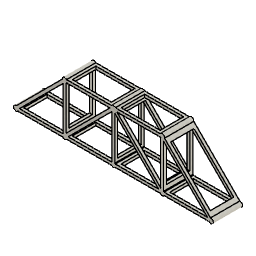
aarav (Autodesk Fusion 360 design; units mm, degrees)
Autodesk Fusion 360 part; units mm, degrees
note: some values were not read from the file. Set by a fixed rule: which sketch regions a step uses.
sketch "Sketch1" plane through (0, 0, 0) normal (0, 1, 0) x (1, 0, 0)
  circle A0 centre (-75, 0) radius 2.5
  line L0 (-75, 0) -> (25, 0) construction
  circle A1 centre (25, 0) radius 2.5
  line L1 (25, 0) -> (25, -50) construction
  line L2 (25, -50) -> (-25, -50) construction
  line L3 (-25, -50) -> (-75, 0) construction
  line L4 (25, -50) -> (-25, 0) construction
  line L5 (-25, -50) -> (-25, 0) construction
  circle A2 centre (-25, -50) radius 2.5
  circle A3 centre (25, -50) radius 2.5
  circle A4 centre (-25, 0) radius 2.5
  line L6 (-23.9393, -48.9393) -> (-73.9393, 1.0607)
  line L7 (-26.0607, -51.0607) -> (-76.0607, -1.0607)
  line L8 (25, -48.5) -> (-25, -48.5)
  line L9 (25, -51.5) -> (-25, -51.5)
  line L10 (23.5, 0) -> (23.5, -50)
  line L11 (26.5, 0) -> (26.5, -50)
  line L12 (23.9393, -51.0607) -> (-26.0607, -1.0607)
  line L13 (26.0607, -48.9393) -> (-23.9393, 1.0607)
  line L14 (-75, -1.5) -> (25, -1.5)
  line L15 (-75, 1.5) -> (25, 1.5)
  line L16 (-23.5, -50) -> (-23.5, 0)
  line L17 (-26.5, -50) -> (-26.5, 0)
  dimension "d1" = 5
  dimension "d2" = 5
  dimension "d3" = 5
  dimension "d4" = 5
  dimension "d5" = 5
  dimension "d6" = 1.5
  dimension "d7" = -1.5
  dimension "d8" = 1.5
  dimension "d9" = -1.5
  dimension "d10" = 1.5
  dimension "d11" = -1.5
  dimension "d12" = -1.5
  dimension "d13" = 1.5
  dimension "d14" = 1.5
  dimension "d15" = -1.5
  dimension "d16" = 1.5
  dimension "d17" = -1.5
  constraint coincident A0.centre L0.start
  constraint horizontal L0
  constraint coincident L0.end A1.centre
  constraint perpendicular L0 L1
  constraint perpendicular L1 L2
  constraint midpoint L0 L4.end
  constraint perpendicular L0 L5
  constraint coincident L2.end L3.start
  constraint coincident L1.end L2.start
  constraint coincident L4.end L5.end
  measures "d1" diameter of A0
  measures "d2" diameter of A1
  measures "d3" diameter of A2
  measures "d4" diameter of A3
  measures "d5" diameter of A4
extrude "Extrude1" add sketch "Sketch1" along normal blind 30 contours A0 | A0 A4 L6 L14 L15 | A0 L6 L14 | A0 A2 L6 L7 L14 L17 | A4 L14 L15 | A4 L15 | A2 L6 L8 | A1 A4 L13 L14 L15 | A4 L14 L17 | A2 A4 L6 L12 L16 L17 | A2 L6 L17 | A2 A3 L8 L9 L12 | A1 L10 L14 | A4 L12 L14 L17 | A2 L6 L8 L16 | A3 L8 L10 | A4 L13 L14 | A1 L10 L14 | A4 L12 L14 L16 | A4 L12 L16 | A2 L8 L16 | A3 L8 L12 | A3 A4 L8 L10 L12 L13 L14 L16 | A4 L14 L16 | A1 A3 L10 L11 L13 | A3 L8 L10 | A3 L10 L13
sketch "Sketch2" plane through (26.5, 0, 0) normal (1, 0, 0) x (0, 1, 0)
  line L0 (0, 48) -> (0, 2)
  line L1 (0, 2) -> (30, 2)
  line L2 (30, 2) -> (30, 48)
  line L3 (30, 48) -> (0, 48)
  line L4 (3, 45) -> (27, 45)
  line L5 (27, 45) -> (27, 5)
  line L6 (27, 5) -> (3, 5)
  line L7 (3, 5) -> (3, 45)
  dimension "d20" = 3
  dimension "d21" = 3
  dimension "d22" = 3
  dimension "d23" = 3
  constraint horizontal L4
  constraint vertical L5
  constraint horizontal L6
  constraint vertical L7
  measures "d20" distance of L3 L4
  measures "d21" distance of L0 L7
  measures "d22" distance of L2 L5
  measures "d23" distance of L1 L6
extrude "Extrude2" cut sketch "Sketch2" against normal blind 3 contours L4 L5 L6 L7
sketch "Sketch3" plane through (-11.4393, 0, 11.4393) normal (0.707107, 0, -0.707107) x (0, 1, 0)
  line L0 (0, 49.4117) -> (0, -14.0563)
  line L1 (0, -14.0563) -> (30, -14.0563)
  line L2 (30, -14.0563) -> (30, 49.4117)
  line L3 (30, 49.4117) -> (0, 49.4117)
  line L4 (3, 46.4117) -> (27, 46.4117)
  line L5 (27, 46.4117) -> (27, -11.0563)
  line L6 (3, -11.0563) -> (3, 46.4117)
  line L7 (3, -11.0563) -> (27, -11.0563)
  dimension "d27" = 3
  dimension "d28" = 3
  dimension "d29" = 3
  dimension "d31" = 3
  constraint horizontal L4
  constraint vertical L5
  constraint vertical L6
  constraint perpendicular L5 L7
  measures "d27" distance of L3 L4
  measures "d28" distance of L2 L5
  measures "d29" distance of L0 L6
  measures "d31" distance of L1 L7
extrude "Extrude3" cut sketch "Sketch3" against normal blind 3 contours L4 L5 L6 L7
sketch "Sketch4" plane through (-23.5, 0, 0) normal (1, 0, 0) x (0, 1, 0)
  line L0 (0, 48) -> (0, 3.6213)
  line L1 (0, 3.6213) -> (30, 3.6213)
  line L2 (30, 3.6213) -> (30, 48)
  line L3 (30, 48) -> (0, 48)
  line L4 (3, 45) -> (3, 6.6213)
  line L5 (3, 6.6213) -> (27, 6.6213)
  line L6 (27, 6.6213) -> (27, 45)
  line L7 (27, 45) -> (3, 45)
  dimension "d34" = 3
  dimension "d35" = 3
  dimension "d36" = 3
  dimension "d37" = 3
  constraint perpendicular L1 L4
  constraint perpendicular L4 L5
  constraint perpendicular L5 L6
  constraint perpendicular L4 L7
  measures "d34" distance of L3 L7
  measures "d35" distance of L0 L4
  measures "d36" distance of L1 L5
  measures "d37" distance of L2 L6
extrude "Extrude4" cut sketch "Sketch4" against normal blind 3 contours L4 L5 L6 L7
sketch "Sketch5" plane through (-36.4393, 0, 36.4393) normal (0.707107, 0, -0.707107) x (0, 1, 0)
  line L0 (0, 14.0563) -> (0, -49.4117)
  line L1 (0, -49.4117) -> (30, -49.4117)
  line L2 (30, -49.4117) -> (30, 14.0563)
  line L3 (30, 14.0563) -> (0, 14.0563)
  line L4 (3, 11.0563) -> (27, 11.0563)
  line L5 (27, 11.0563) -> (27, -46.4117)
  line L6 (3, -46.4117) -> (27, -46.4117)
  line L7 (3, 11.0563) -> (3, -46.4117)
  dimension "d41" = 3
  dimension "d42" = 3
  dimension "d43" = 3
  dimension "d44" = 3
  constraint parallel L3 L4
  constraint perpendicular L4 L5
  constraint coincident L5 L6.end
  constraint perpendicular L5 L6
  constraint coincident L6 L7.end
  constraint perpendicular L6 L7
  measures "d41" distance of L0 L7
  measures "d42" distance of L3 L4
  measures "d43" distance of L2 L5
  measures "d44" distance of L1 L6
extrude "Extrude5" cut sketch "Sketch5" against normal blind 3 contours L4 L5 L6 L7
ref_plane "WorkPlane1" through (25, 15, 24.1893) normal (-1, 0, 0) x (0, 0, 1)
sketch "Sketch6" plane through (0, 0, 51.5) normal (0, 0, 1) x (-1, 0, 0)
  line L0 (23, 0) -> (-23, 0)
  line L1 (-23, 0) -> (-23, -30)
  line L2 (-23, -30) -> (23, -30)
  line L3 (23, -30) -> (23, 0)
  line L4 (20, -27) -> (-20, -27)
  line L5 (-20, -27) -> (-20, -3)
  line L6 (-20, -3) -> (20, -3)
  line L7 (20, -3) -> (20, -27)
  dimension "d47" = 3
  dimension "d48" = 3
  dimension "d49" = 3
  dimension "d50" = 3
  constraint horizontal L4
  constraint vertical L5
  constraint horizontal L6
  constraint vertical L7
  measures "d47" distance of L2 L4
  measures "d48" distance of L3 L7
  measures "d49" distance of L0 L6
  measures "d50" distance of L1 L5
extrude "Extrude6" cut sketch "Sketch6" against normal blind 3 contours L4 L5 L6 L7
sketch "Sketch7" plane through (0, 0, -1.5) normal (0, 0, -1) x (1, 0, 0)
  line L0 (23, 0) -> (-23, 0)
  line L1 (-23, 0) -> (-23, -30)
  line L2 (-23, -30) -> (23, -30)
  line L3 (23, -30) -> (23, 0)
  line L4 (20, -27) -> (-20, -27)
  line L5 (-20, -27) -> (-20, -3)
  line L6 (-20, -3) -> (20, -3)
  line L7 (20, -3) -> (20, -27)
  dimension "d53" = 3
  dimension "d54" = 3
  dimension "d55" = 3
  dimension "d56" = 3
  constraint horizontal L4
  constraint vertical L5
  constraint horizontal L6
  constraint vertical L7
  measures "d53" distance of L2 L4
  measures "d54" distance of L3 L7
  measures "d55" distance of L0 L6
  measures "d56" distance of L1 L5
extrude "Extrude7" cut sketch "Sketch7" against normal blind 3 contours L4 L5 L6 L7
sketch "Sketch8" plane through (0, 0, -1.5) normal (0, 0, -1) x (1, 0, 0)
  line L0 (-27, 0) -> (-73, 0)
  line L1 (-73, 0) -> (-73, -30)
  line L2 (-73, -30) -> (-27, -30)
  line L3 (-27, -30) -> (-27, 0)
  line L4 (-30, -27) -> (-70, -27)
  line L5 (-70, -27) -> (-70, -3)
  line L6 (-70, -3) -> (-30, -3)
  line L7 (-30, -3) -> (-30, -27)
  dimension "d59" = 3
  dimension "d60" = 3
  dimension "d61" = 3
  dimension "d62" = 3
  constraint horizontal L4
  constraint vertical L5
  constraint horizontal L6
  constraint vertical L7
  measures "d59" distance of L2 L4
  measures "d60" distance of L3 L7
  measures "d61" distance of L0 L6
  measures "d62" distance of L1 L5
extrude "Extrude8" cut sketch "Sketch8" against normal blind 3 contours L4 L5 L6 L7
mirror "Mirror1" about plane through (25, 15, 24.1893) normal (-1, 0, 0) of bodies 1 merged
